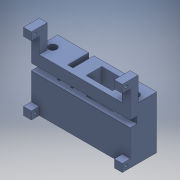
# Autodesk Inventor part: SupportPlateau
Saved by Autodesk Inventor 2017 SP1 (Build 210196100, 196)
## iProperties
Created: 2017-10-26
Part Number: SupportPlateau
Material: PC/ABS Plastic
Document SubType Name: Modeling
Designer: Biscuit
Density: 0.357273 g/cm^3
Appearance: Rubber - Blue
Author: Biscuit
Autodesk Inventor part; units mm, degrees
ref_plane "YZ Plane" through (0, 0, 0) normal (1, 0, 0) x (0, 1, 0)
ref_plane "XZ Plane" through (0, 0, 0) normal (0, 1, 0) x (-1, 0, 0)
ref_plane "XY Plane" through (0, 0, 0) normal (0, 0, 1) x (1, 0, 0)
sketch "Sketch3" plane through (0, 0, 0) normal (0, 0, 1) x (1, 0, 0)
  line L0 (0, 0) -> (75, 0)
  line L1 (75, 0) -> (75, 20)
  line L2 (75, 20) -> (0, 20)
  line L3 (0, 20) -> (0, 0)
  circle A0 centre (6.25, 10) radius 3
  circle A1 centre (68.75, 10) radius 3
  line L4 (37.5, 16) -> (57.5, 16)
  line L5 (57.5, 16) -> (57.5, 4)
  line L6 (57.5, 4) -> (37.5, 4)
  line L7 (37.5, 4) -> (37.5, 16)
  dimension "d19" = 20
  dimension "d20" = 75
  dimension "d21" = 6
  dimension "d22" = 6
  dimension "d23" = 10
  dimension "d24" = 10
  dimension "d25" = 62.5
  dimension "d26" = 6.25
  dimension "d30" = 12
  dimension "d31" = 20
  dimension "d32" = 4
  dimension "d33" = 17.5
  constraints: 16 end point, 4 parallel, 2 centre point, 2 horizontal, 2 perpendicular
  measures "d19" distance of L2.end L0.start
  measures "d20" distance of L1.end L2.end
  measures "d21" diameter of A0
  measures "d22" diameter of A1
  measures "d23" distance from line of L0 A0.centre
  measures "d24" distance from line of L0 A1.centre
  measures "d25" distance of A1.centre A0.centre
  measures "d26" distance from line of L3 A0.centre
  measures "d30" distance of L6.end L4.start
  measures "d31" distance of L4.start L4.end
  measures "d32" distance between parallel lines of L2 L4
  measures "d33" distance between parallel lines of L1 L5
extrude "Extrusion3" add sketch "Sketch3" along normal blind 40
sketch "Sketch4" plane through (0, 20, 0) normal (0, 1, 0) x (1, 0, 0)
  line L0 (0, 0) -> (75, 0) projected
  line L1 (27.5, -40) -> (27.5, -20)
  line L2 (27.5, -20) -> (15.5, -20)
  line L3 (15.5, -20) -> (15.5, -32)
  line L4 (15.5, -32) -> (23.5, -32)
  line L5 (23.5, -32) -> (23.5, -40)
  line L6 (17.5, -22) -> (25.5, -22)
  line L7 (25.5, -22) -> (25.5, -30)
  line L8 (25.5, -30) -> (17.5, -30)
  line L9 (17.5, -30) -> (17.5, -22)
  line L10 (23.5, -40) -> (27.5, -40)
  line L11 (0, 0) -> (0, -40) projected
  line L12 (75, -40) -> (0, -40) projected
  line L13 (75, 0) -> (75, -40) projected
  line L14 (27.5, 0) -> (27.5, -20)
  line L15 (15.5, -20) -> (15.5, -8)
  line L16 (15.5, -8) -> (23.5, -8)
  line L17 (23.5, -8) -> (23.5, 0)
  line L18 (17.5, -18) -> (25.5, -18)
  line L19 (25.5, -18) -> (25.5, -10)
  line L20 (25.5, -10) -> (17.5, -10)
  line L21 (17.5, -10) -> (17.5, -18)
  line L22 (23.5, 0) -> (27.5, 0)
  dimension "d34" = 2
  dimension "d35" = 2
  dimension "d36" = 2
  dimension "d37" = 2
  dimension "d38" = 4
  dimension "d39" = 32
  dimension "d40" = 8
  dimension "d41" = 8
  dimension "d42" = 27.5
  dimension "d43" = 40
  constraints: 38 end point, 8 symmetric about line, 5 perpendicular, 2 parallel
  measures "d34" distance between parallel lines of L1 L7
  measures "d35" distance between parallel lines of L3 L9
  measures "d36" distance between parallel lines of L2 L6
  measures "d37" distance between parallel lines of L4 L8
  measures "d38" distance between parallel lines of L1 L5
  measures "d39" distance between parallel lines of L0 L4
  measures "d40" distance between parallel lines of L7 L9
  measures "d41" distance between parallel lines of L8 L6
  measures "d42" distance between parallel lines of L11 L1
  measures "d43" distance between parallel lines of L0 L12
extrude "Extrusion4" cut sketch "Sketch4" against normal blind 16 contours L0 L14 L2 L15 L16 L17 | L5 L4 L3 L2 L1 L10
sketch "Sketch5" plane through (0, 0, 0) normal (0, -1, 0) x (1, 0, 0)
  line L0 (0, 0) -> (75, 0) projected
  line L1 (0, 40) -> (75, 40) projected
  line L2 (75, 0) -> (75, 40) projected
  line L3 (0, 0) -> (0, 40) projected
  line L4 (0, 40) -> (6, 40)
  line L5 (6, 40) -> (6, 58)
  line L6 (6, 58) -> (0, 58)
  line L7 (0, 58) -> (0, 40)
  line L8 (75, 40) -> (69, 40)
  line L9 (69, 40) -> (69, 58)
  line L10 (69, 58) -> (75, 58)
  line L11 (75, 58) -> (75, 40)
  dimension "d46" = 40
  dimension "d47" = 75
  dimension "d48" = 6
  dimension "d49" = 18
  dimension "d79" = 6
  dimension "d80" = 18
  constraints: 16 end point, 4 parallel, 2 horizontal, 2 perpendicular
  measures "d46" distance between parallel lines of L0 L1
  measures "d47" distance between parallel lines of L2 L3
  measures "d48" distance of L5.end L6.end
  measures "d49" distance of L6.end L1.start
  measures "d79" distance of L9.end L10.end
  measures "d80" distance of L8.end L9.end
extrude "Extrusion5" add sketch "Sketch5" against normal blind 6 contours L7 L6 L5 L1 | L1 L9 L10 L11
sketch "Sketch6" plane through (0, 0, 0) normal (0, -1, 0) x (1, 0, 0)
  line L0 (6, 58) -> (0, 58) projected
  line L1 (0, 40) -> (0, 58) projected
  line L2 (6, 58) -> (0, 58)
  line L3 (0, 58) -> (0, 52)
  line L4 (0, 52) -> (6, 52)
  line L5 (6, 52) -> (6, 58)
  line L6 (0, 0) -> (0, 40) projected
  line L7 (0, 0) -> (6, 0)
  line L8 (6, 0) -> (6, 6)
  line L9 (6, 6) -> (0, 6)
  line L10 (0, 6) -> (0, 0)
  line L11 (75, 0) -> (75, 40) projected
  line L12 (75, 0) -> (69, 0)
  line L13 (69, 0) -> (69, 6)
  line L14 (69, 6) -> (75, 6)
  line L15 (75, 6) -> (75, 0)
  line L16 (75, 0) -> (75, 58) projected
  line L17 (69, 40) -> (69, 58) projected
  line L18 (75, 58) -> (69, 58)
  line L19 (69, 58) -> (69, 52)
  line L20 (69, 52) -> (75, 52)
  line L21 (75, 52) -> (75, 58)
  dimension "d52" = 6
  dimension "d53" = 6
  dimension "d54" = 6
  dimension "d81" = 6
  dimension "d82" = 6
  dimension "d83" = 6
  constraints: 32 end point, 8 parallel, 4 horizontal, 4 perpendicular, 2 point on line
  measures "d52" distance between parallel lines of L0 L4
  measures "d53" distance of L8.end L9.end
  measures "d54" distance of L7.end L8.end
  measures "d81" distance of L18.end L19.end
  measures "d82" distance of L13.end L14.end
  measures "d83" distance of L12.end L13.end
extrude "Extrusion6" add sketch "Sketch6" along normal blind 6
sketch "Sketch7" plane through (0, 6, 58) normal (0, 0, 1) x (1, 0, 0)
  circle A0 centre (3, -9) radius 1
  line L0 (0, 0) -> (0, -12) projected
  line L1 (6, 0) -> (6, -12) projected
  line L2 (6, -12) -> (0, -12) projected
  line L3 (6, -6) -> (69, -6) projected
  line L4 (75, 0) -> (75, -12) projected
  line L5 (69, 0) -> (75, 0) projected
  line L6 (69, 0) -> (69, -12) projected
  line L7 (75, -12) -> (69, -12) projected
  circle A1 centre (72, -9) radius 1
  point P0 (0, -6)
  point P1 (75, -6)
  dimension "d57" = 2
  dimension "d58" = 6
  dimension "d59" = 6
  dimension "d60" = 3
  dimension "d61" = 3
  dimension "d84" = 2
  dimension "d85" = 3
  dimension "d86" = 3
  constraints: 2 centre point
  measures "d57" diameter of A0
  measures "d58" distance between parallel lines of L0 L1
  measures "d59" distance between parallel lines of L2 L3
  measures "d60" distance from line of L2 A0.centre
  measures "d61" distance from line of L1 A0.centre
  measures "d84" diameter of A1
  measures "d85" distance from line of L7 A1.centre
  measures "d86" distance from line of L4 A1.centre
extrude "Extrusion7" [suppressed]
sketch "Sketch8" plane through (75, 20, 40) normal (0, 1, 0) x (1, 0, 0)
  circle A0 centre (-15.75, 12) radius 1
  line L0 (-47.5, 40) -> (-47.5, 0) projected
  line L1 (0, 0) -> (-47.5, 0) projected
  line L2 (0, 40) -> (0, 0) projected
  line L3 (0, 40) -> (-47.5, 40) projected
  circle A1 centre (-31.75, 12) radius 1
  circle A2 centre (-15.75, 28) radius 1
  circle A3 centre (-31.75, 28) radius 1
  point P0 (-75, 40)
  dimension "d64" = 2
  dimension "d67" = 16
  dimension "d70" = 16
  dimension "d73" = 15.75
  dimension "d74" = 47.5
  dimension "d75" = 40
  dimension "d76" = 12
  constraints: 4 centre point, 1 horizontal, 1 vertical, 6 other
  measures "d64" diameter of A0
  measures "d67" distance of A0.centre A1.centre
  measures "d70" distance of A0.centre A2.centre
  measures "d73" distance from line of L2 A0.centre
  measures "d74" distance of L1.start L0.end
  measures "d75" distance of L2.start L1.start
  measures "d76" distance from line of L1 A0.centre
extrude "Extrusion8" cut sketch "Sketch8" against normal blind 5 contours A0 | A1 | A2 | A3
sketch "Esquisse9" plane through (75, 20, 40) normal (1, 0, 0) x (0, 0, -1)
  circle A0 centre (-15, -23) radius 1
  circle A1 centre (37, -23) radius 1
  line L0 (40, 0) -> (40, -26) projected
  line L1 (40, 0) -> (0, 0) projected
  line L2 (0, -14) -> (0, 0) projected
  line L3 (-18, -14) -> (0, -14) projected
  line L4 (-18, -14) -> (-18, -26) projected
  line L5 (-12, -26) -> (-18, -26) projected
  line L6 (-12, -20) -> (-12, -26) projected
  line L7 (34, -20) -> (-12, -20) projected
  line L8 (34, -20) -> (34, -26) projected
  line L9 (40, -26) -> (34, -26) projected
  point P0 (40, -20)
  dimension "d87" = 2
  dimension "d88" = 2
  dimension "d89" = 6
  dimension "d90" = 6
  dimension "d91" = 3
  dimension "d92" = 3
  dimension "d93" = 6
  dimension "d94" = 6
  dimension "d95" = 3
  dimension "d96" = 3
  constraints: 2 centre point
  measures "d87" diameter of A0
  measures "d88" diameter of A1
  measures "d89" distance of L5.start L4.end
  measures "d90" distance of L6.start L5.start
  measures "d91" distance from line of L6 A0.centre
  measures "d92" distance from line of L5 A0.centre
  measures "d93" distance of L0.end L8.end
  measures "d94" distance of L7.start L8.end
  measures "d95" distance from line of L0 A1.centre
  measures "d96" distance from line of L9 A1.centre
extrude "Extrusion9" cut sketch "Esquisse9" against normal through all contours A0 | A1
sketch "Esquisse10" plane through (6, 0, 40) normal (0, -1, 0) x (1, 0, 0)
  line L0 (69, 12) -> (63, 12) projected
  line L1 (63, 12) -> (63, 0) projected
  line L2 (0, 0) -> (63, 0) projected
  line L3 (0, 0) -> (0, 12) projected
  line L4 (0, 12) -> (-6, 12) projected
  line L5 (-6, -34) -> (-6, 12) projected
  line L6 (-6, -34) -> (0, -34) projected
  line L7 (0, -34) -> (0, -40) projected
  line L8 (0, -40) -> (63, -40) projected
  line L9 (63, -40) -> (63, -34) projected
  line L10 (63, -34) -> (69, -34) projected
  line L11 (69, -34) -> (69, 12) projected
  line L12 (69, -34) -> (69, 12) projected
  line L13 (-6, -8.5) -> (69, -8.5)
  line L14 (69, -8.5) -> (69, -13.5)
  line L15 (69, -13.5) -> (-6, -13.5)
  line L16 (-6, -13.5) -> (-6, -8.5)
  point P0 (-6, -40)
  dimension "d99" = 5
  dimension "d100" = 46
  dimension "d101" = 20.5
  constraints: 8 end point, 2 parallel, 2 point on line, 1 horizontal, 1 perpendicular
  measures "d99" distance between parallel lines of L15 L13
  measures "d100" distance between parallel lines of L4 L6
  measures "d101" distance between parallel lines of L4 L13
extrude "Extrusion10" cut sketch "Esquisse10" against normal blind 5 contours L11 L15 L5 L13
equation "\"d22\" = d21"
equation "\"d23\" = 0.5 * d19"
equation "\"d24\" = 0.5 * d19"
equation "\"d26\" = 0.5 * d20 - 0.5 * d25"
equation "\"d32\" = 0.5 * d19 - 0.5 * d30"
equation "\"d33\" = 0.5 * d20 - d31"
equation "\"d35\" = d34"
equation "\"d36\" = d34"
equation "\"d37\" = d34"
equation "\"d38\" = 2 * d34"
equation "\"d40\" = 4 * d34"
equation "\"d41\" = 4 * d34"
equation "\"d79\" = d48"
equation "\"d80\" = d49"
equation "\"d81\" = d52"
equation "\"d82\" = d53"
equation "\"d83\" = d54"
equation "\"d60\" = 0.5 * d59"
equation "\"d61\" = 0.5 * d58"
equation "\"d84\" = d57"
equation "\"d85\" = d60"
equation "\"d86\" = d61"
equation "\"d73\" = 0.5 * d74 - 0.5 * d67"
equation "\"d76\" = 0.5 * d75 - 0.5 * d70"
equation "\"d88\" = d87"
equation "\"d91\" = 0.5 * d89"
equation "\"d92\" = 0.5 * d90"
equation "\"d95\" = 0.5 * d93"
equation "\"d96\" = 0.5 * d94"
equation "\"d101\" = 0.5 * d100 - 0.5 * d99"
body "Solid2"
